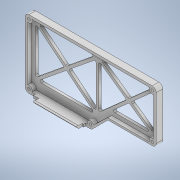
# Autodesk Inventor part: bottom rev3
Saved by Autodesk Inventor 2021 (Build 250183000, 183)
## iProperties
Created: 2024-09-17
Part Number: bottom rev3
Material: Generic
Document SubType Name: Modeling
Designer: Toby
Density: 1 g/cm^3
Appearance: Default
Author: Toby
Autodesk Inventor part; units mm, degrees
ref_plane "YZ Plane" through (0, 0, 0) normal (1, 0, 0) x (0, 1, 0)
ref_plane "XZ Plane" through (0, 0, 0) normal (0, 1, 0) x (-1, 0, 0)
ref_plane "XY Plane" through (0, 0, 0) normal (0, 0, 1) x (1, 0, 0)
sketch "Sketch1" plane through (0, 0, 0) normal (0, 0, 1) x (1, 0, 0)
  line L0 (-50, 26) -> (50, 26)
  line L1 (50, 26) -> (50, -26)
  line L2 (50, -26) -> (-50, -26)
  line L3 (-50, -26) -> (-50, 26)
  point P0 (0, 0)
  dimension "d0" = 52
  dimension "d1" = 100
  dimension "d2" = 26
  dimension "d3" = 50
  constraints: 8 end point, 2 parallel, 1 horizontal, 1 perpendicular
  measures "d0" distance of L2.end L0.start
  measures "d1" distance of L0.start L0.end
  measures "d2" distance from line of point (0, 0) L0
  measures "d3" distance from line of point (0, 0) L3
extrude "Extrusion1" add sketch "Sketch1" along normal blind 2
sketch "Sketch2" plane through (0, 0, 2) normal (0, 0, 1) x (1, 0, 0)
  line L0 (-50, 26) -> (-50, -26) projected
  line L1 (-50, -26) -> (50, -26) projected
  circle A0 centre (-47, 23) radius 1
  circle A1 centre (-47, 23) radius 2.5
  circle A2 centre (-47, -23) radius 1
  circle A3 centre (-47, -23) radius 2.5
  circle A4 centre (0, -23) radius 1
  circle A5 centre (0, -23) radius 2.5
  circle A6 centre (47, 23) radius 1
  circle A7 centre (47, 23) radius 2.5
  circle A8 centre (47, -11) radius 1
  circle A9 centre (47, -11) radius 2.5
  point P0 (0, 0)
  dimension "d6" = 3
  dimension "d7" = 3
  dimension "d8" = 50
  dimension "d9" = 3
  dimension "d10" = 97
  dimension "d11" = 15
  dimension "d12" = 3
  dimension "d13" = 49
  dimension "d14" = 97
  dimension "d15" = 49
  dimension "d16" = 2
  dimension "d17" = 5
  dimension "d18" = 2
  dimension "d19" = 5
  dimension "d20" = 2
  dimension "d21" = 5
  dimension "d22" = 2
  dimension "d23" = 5
  dimension "d24" = 2
  dimension "d25" = 5
  constraints: 10 centre point, 10 coincident
  measures "d6" distance from line of L0 point (-47, -23)
  measures "d7" distance from line of L1 point (-47, -23)
  measures "d8" distance from line of L0 point (0, -23)
  measures "d9" distance from line of L1 point (0, -23)
  measures "d10" distance from line of L0 point (47, -11)
  measures "d11" distance from line of L1 point (47, -11)
  measures "d12" distance from line of L0 point (-47, 23)
  measures "d13" distance from line of L1 point (-47, 23)
  measures "d14" distance from line of L0 point (47, 23)
  measures "d15" distance from line of L1 point (47, 23)
  measures "d16" diameter of A0
  measures "d17" diameter of A1
  measures "d18" diameter of A2
  measures "d19" diameter of A3
  measures "d20" diameter of A4
  measures "d21" diameter of A5
  measures "d22" diameter of A6
  measures "d23" diameter of A7
  measures "d24" diameter of A8
  measures "d25" diameter of A9
extrude "Extrusion2" add sketch "Sketch2" along normal blind 3
sketch "Sketch3" plane through (0, 0, 0) normal (0, 0, -1) x (-1, 0, 0)
  circle A0 centre (-47, 23) radius 1 projected
  circle A1 centre (47, 23) radius 1 projected
  circle A2 centre (47, -23) radius 1 projected
  circle A3 centre (0, -23) radius 1 projected
  circle A4 centre (-47, -11) radius 1 projected
  point P0 (0, 0)
  constraints: 5 coincident
hole "Hole1" at (47, 23, 0) at (-47, 23, 0) at (-47, -23, 0) at (0, -23, 0) at (47, -11, 0) direction (0, 0, 1) diameter 2 depth 10 tip angle 118 countersink diameter 5 countersink angle 90
sketch "Sketch4" plane through (0, 0, 2) normal (0, 0, 1) x (1, 0, 0)
  line L0 (50, -26) -> (50, 26) projected
  line L1 (50, -26) -> (13.1, -26)
  line L2 (13.1, -26) -> (13.1, -13.5)
  line L3 (13.1, -13.5) -> (50, -13.5)
  line L4 (50, -13.5) -> (50, -26)
  line L5 (-50, 26) -> (-50, -26) projected
  point P0 (0, 0)
  dimension "d35" = 12.5
  dimension "d36" = 63.1
  constraints: 8 end point, 2 parallel, 1 horizontal, 1 perpendicular
  measures "d35" distance between parallel lines of L1 L3
  measures "d36" distance between parallel lines of L5 L2
extrude "Extrusion3" cut sketch "Sketch4" against normal blind 3
sketch "Sketch5" plane through (0, 0, 2) normal (0, 0, 1) x (1, 0, 0)
  line L0 (-50, -26) -> (13.1, -26) projected
  line L1 (-50, 26) -> (-50, -26) projected
  line L2 (13.1, -13.5) -> (0.673, -26)
  line L3 (0.673, -26) -> (13.1, -26)
  line L4 (13.1, -26) -> (13.1, -13.5) projected
  line L5 (13.1, -13.5) -> (13.1, -26)
  point P0 (0, 0)
  dimension "d39" = 50.673
  constraints: 6 end point, 1 horizontal, 1 point on line, 1 vertical
  measures "d39" distance from line of L1 L2.end
extrude "Extrusion4" cut sketch "Sketch5" against normal blind 3
sketch "Sketch6" plane through (0, 0, 2) normal (0, 0, 1) x (1, 0, 0)
  line L0 (-50, 26) -> (-50, -26) projected
  line L1 (-50, -26) -> (0.673, -26) projected
  line L2 (-50, 26) -> (-48, 26)
  line L3 (-48, 26) -> (-48, -26)
  line L4 (-48, -26) -> (-50, -26)
  line L5 (-50, -26) -> (-50, 26)
  line L6 (50, -13.5) -> (50, 26) projected
  line L7 (-48, 26) -> (50, 26)
  line L8 (50, 26) -> (50, 24)
  line L9 (50, 24) -> (-48, 24)
  line L10 (-48, 24) -> (-48, 26)
  circle A0 centre (47, -11) radius 2.5 projected
  line L11 (50, 24) -> (48, 24)
  line L12 (48, 24) -> (48, -13.2913)
  line L13 (48, -13.2913) -> (50, -13.2913)
  line L14 (50, -13.2913) -> (50, 24)
  circle A1 centre (0, -23) radius 1 projected
  line L15 (-48, -26) -> (0, -26)
  line L16 (0, -26) -> (0, -24)
  line L17 (0, -24) -> (-48, -24)
  line L18 (-48, -24) -> (-48, -26)
  line L19 (50, -13.5) -> (47, -13.5) projected
  line L20 (50, -13.2913) -> (48, -13.2913)
  line L21 (48, -13.2913) -> (48, -13.5)
  line L22 (48, -13.5) -> (50, -13.5)
  line L23 (50, -13.5) -> (50, -13.2913)
  line L24 (0.673, -26) -> (13.1, -13.5) projected
  line L25 (13.1, -13.5) -> (50, -13.5)
  line L26 (50, -13.5) -> (50, -12)
  line L27 (50, -12) -> (13.1, -12)
  line L28 (13.1, -12) -> (13.1, -13.5)
  line L29 (0, -26) -> (0.673, -26)
  line L30 (0.673, -26) -> (13.1, -13.5)
  line L31 (13.1, -12) -> (13.1, -13.5)
  line L32 (13.1, -12) -> (0.6867, -23.7269)
  line L33 (0.6867, -23.7269) -> (0.6867, -24)
  line L34 (0.6867, -24) -> (0, -24)
  point P0 (0, 0)
  point P1 (44.7087, -12)
  point P2 (-48, 24)
  point P3 (48, -8.7087)
  dimension "d42" = 2
  dimension "d43" = 2
  dimension "d44" = 2
  dimension "d45" = 1.5
  constraints: 60 end point, 13 parallel, 8 perpendicular, 6 horizontal, 6 point on line, 3 point on circle, 2 tangent, 1 collinear
  measures "d42" distance of L3.end L4.end
  measures "d43" distance of L7.end L8.end
  measures "d44" distance of L13.end L12.end
  measures "d45" distance of L26.end L25.end
extrude "Extrusion5" add sketch "Sketch6" along normal blind 3 contours L2 L3 L1 L0 | L7 L6 L9 L3 | L3 L17 L16 L1 | L16 L34 L33 L32 L28 L24 L1 | L9 L6 L27 A0 L12 | L6 L13 A0 L27 | L28 L27 A0 L25 | L6 L19 L21 L13 | A0 L21 L19
fillet "Fillet1" radius 3 4 edges at (50, 26, 2.5) (50, -13.5, 2.5) (-50, -26, 2.5) (-50, 26, 2.5)
sketch "Sketch7" plane through (0, 0, 5) normal (0, 0, 1) x (1, 0, 0)
  line L0 (-47, -26) -> (0.673, -26) projected
  line L1 (-42.4, -26) -> (-3.6, -26)
  line L2 (-3.6, -26) -> (-3.6, -19.3)
  line L3 (-3.6, -19.3) -> (-42.4, -19.3)
  line L4 (-42.4, -19.3) -> (-42.4, -26)
  line L5 (-50, 23) -> (-50, -23) projected
  point P0 (0, 0)
  dimension "d49" = 7.6
  dimension "d50" = 46.4
  dimension "d51" = 6.7
  constraints: 8 end point, 2 parallel, 1 horizontal, 1 perpendicular, 1 point on line
  measures "d49" distance between parallel lines of L5 L4
  measures "d50" distance between parallel lines of L5 L2
  measures "d51" distance between parallel lines of L0 L3
extrude "Extrusion6" cut sketch "Sketch7" against normal blind 3
sketch "Sketch8" plane through (0, 0, 2) normal (0, 0, 1) x (1, 0, 0)
  line L0 (-47, -26) -> (-42.4, -26) projected
  line L1 (-42.4, -26) -> (-37.4, -26)
  line L2 (-37.4, -26) -> (-37.4, -24)
  line L3 (-37.4, -24) -> (-42.4, -24)
  line L4 (-42.4, -24) -> (-42.4, -26)
  point P0 (0, 0)
  dimension "d54" = 5
  dimension "d55" = 2
  constraints: 8 end point, 2 parallel, 1 horizontal, 1 perpendicular
  measures "d54" distance of L2.end L3.end
  measures "d55" distance between parallel lines of L1 L3
extrude "Extrusion7" add sketch "Sketch8" along normal blind 12
sketch "Sketch9" plane through (0, 0, 2) normal (0, 0, 1) x (1, 0, 0)
  line L0 (-39.4, -21.4) -> (-28.4, -21.4)
  line L1 (-28.4, -21.4) -> (-28.4, -22.6)
  line L2 (-28.4, -22.6) -> (-39.4, -22.6)
  line L3 (-39.4, -22.6) -> (-39.4, -21.4)
  line L4 (-37.4, -24) -> (-42.4, -24) projected
  line L5 (-42.4, -24) -> (-42.4, -26) projected
  line L6 (-15.6, -21.4) -> (-3.6, -21.4)
  line L7 (-3.6, -21.4) -> (-3.6, -22.6)
  line L8 (-3.6, -22.6) -> (-15.6, -22.6)
  line L9 (-15.6, -22.6) -> (-15.6, -21.4)
  line L10 (-3.6, -24) -> (-3.6, -26) projected
  line L11 (-2.2913, -24) -> (-3.6, -24) projected
  point P0 (0, 0)
  dimension "d58" = 1.4
  dimension "d59" = 1.2
  dimension "d60" = 3
  dimension "d61" = 14
  dimension "d62" = 1.2
  dimension "d63" = 1.4
  dimension "d64" = 12
  constraints: 16 end point, 4 parallel, 2 horizontal, 2 perpendicular, 1 collinear
  measures "d58" distance between parallel lines of L4 L2
  measures "d59" distance between parallel lines of L2 L0
  measures "d60" distance between parallel lines of L5 L3
  measures "d61" distance between parallel lines of L5 L1
  measures "d62" distance between parallel lines of L8 L6
  measures "d63" distance between parallel lines of L11 L8
  measures "d64" distance of L6.start L6.end
extrude "Extrusion8" add sketch "Sketch9" along normal blind 3
chamfer "Chamfer1" distance 1 angle 45 2 edges at (-33.9, -21.4, 2) (-9.6, -21.4, 2)
sketch "Sketch10" plane through (0, 0, 2) normal (0, 0, 1) x (1, 0, 0)
  line L0 (-3.6, -22.6) -> (-3.6, -21.4) projected
  line L1 (-3.6, -24) -> (-2.2913, -24) projected
  line L2 (-3.6, -21.4) -> (-2.4, -21.4)
  line L3 (-2.4, -21.4) -> (-2.4, -24)
  line L4 (-2.4, -24) -> (-3.6, -24)
  line L5 (-3.6, -24) -> (-3.6, -21.4)
  line L6 (-2.4, -24) -> (-2.1404, -24)
  line L7 (-2.1404, -24) -> (-2.1404, -23.6677)
  line L8 (-2.1404, -23.6677) -> (-2.4, -23.6677)
  line L9 (-2.4, -23.6677) -> (-2.4, -24)
  point P0 (0, 0)
  dimension "d70" = 1.2
  constraints: 16 end point, 4 parallel, 2 horizontal, 2 perpendicular, 1 point on line
  measures "d70" distance of L3.end L4.end
extrude "Extrusion9" add sketch "Sketch10" along normal blind 3
fillet "Fillet2" radius 1 1 edges at (-2.4, -21.4, 3.5)
sketch "Sketch12" plane through (0.673, -26, 0) normal (0, -1, 0) x (1, 0, 0)
  line L0 (-43.073, 5) -> (-43.073, 14) projected
  line L1 (-43.073, 14) -> (-38.073, 14)
  line L2 (-38.073, 14) -> (-38.073, 5)
  line L3 (-38.073, 5) -> (-43.073, 5)
  line L4 (-43.073, 5) -> (-43.073, 14)
  line L5 (-38.073, 2) -> (-38.073, 14) projected
  line L6 (-40.073, 5) -> (-29.073, 5) projected
  point P0 (-0.673, 0)
  constraints: 8 end point, 2 collinear, 2 parallel, 1 horizontal, 1 perpendicular
extrude "Extrusion11" cut sketch "Sketch12" against normal blind 3
sketch "Sketch13" plane through (0, 0, 2) normal (0, 0, 1) x (1, 0, 0)
  line L0 (-45, 21) -> (45, 21)
  line L1 (45, 21) -> (45, -9)
  line L2 (45, -9) -> (-45, -9)
  line L3 (-45, -9) -> (-45, 21)
  line L4 (-45, -9) -> (2, -9)
  line L5 (2, -9) -> (2, -17.4)
  line L6 (2, -17.4) -> (-45, -17.4)
  line L7 (-45, -17.4) -> (-45, -9)
  line L8 (-44.7087, 24) -> (44.7087, 24) projected
  line L9 (-48, -20.7087) -> (-48, 20.7087) projected
  line L10 (48, 20.7087) -> (48, -8.7087) projected
  line L11 (44.7087, 24) -> (-44.7087, 24) projected
  line L12 (48, -8.7087) -> (48, 20.7087) projected
  line L13 (44, 24) -> (48, 24)
  line L14 (48, 24) -> (48, 20)
  line L15 (48, 20) -> (44, 20)
  line L16 (44, 20) -> (44, 24)
  circle A0 centre (47, 23) radius 1 projected
  line L17 (44.7087, -12) -> (13.1, -12) projected
  line L18 (-28.4, -20.4) -> (-39.4, -20.4) projected
  line L19 (50, -10.5) -> (50, 23) projected
  point P0 (0, 0)
  point P1 (48, 24)
  point P2 (45, 20)
  point P3 (44, 21)
  dimension "d79" = 3
  dimension "d80" = 3
  dimension "d81" = 3
  dimension "d82" = 3
  dimension "d83" = 3
  dimension "d84" = 3
  dimension "d85" = 3
  dimension "d86" = 48
  constraints: 24 end point, 6 parallel, 3 horizontal, 3 perpendicular, 2 point on line
  measures "d79" distance between parallel lines of L0 L8
  measures "d80" distance between parallel lines of L9 L3
  measures "d81" distance between parallel lines of L10 L1
  measures "d82" distance from line of A0.centre L16
  measures "d83" distance from line of L15 A0.centre
  measures "d84" distance between parallel lines of L17 L2
  measures "d85" distance between parallel lines of L18 L6
  measures "d86" distance between parallel lines of L19 L5
extrude "Extrusion12" cut sketch "Sketch13" against normal blind 2 contours L0 L16 L15 L1 L2 L3 | L2 L5 L6 L7
chamfer "Chamfer2" distance 8.4 angle 45 1 edges at (2, -9, 1)
sketch "Sketch14" plane through (0, 0, 5) normal (0, 0, 1) x (1, 0, 0)
  line L0 (-28.4, -20.4) -> (-39.4, -20.4) projected
  line L1 (-39.4, -20.4) -> (-2.4, -20.4)
  line L2 (-2.4, -20.4) -> (-2.4, -24)
  line L3 (-2.4, -24) -> (-39.4, -24)
  line L4 (-39.4, -24) -> (-39.4, -20.4)
  line L5 (-37.4, -24) -> (-44.7087, -24) projected
  line L6 (-3.6, -22.6) -> (-3.6, -26) projected
  point P0 (0, 0)
  dimension "d92" = 1.2
  constraints: 8 end point, 2 parallel, 1 collinear, 1 horizontal, 1 perpendicular
  measures "d92" distance between parallel lines of L6 L2
extrude "Extrusion13" cut sketch "Sketch14" against normal blind 3
sketch "Sketch15" plane through (0, 0, 5) normal (0, 0, 1) x (1, 0, 0)
  line L0 (-44.7087, -24) -> (-37.4, -24) projected
  line L1 (-42.4, -24) -> (-3.6, -24)
  line L2 (-3.6, -24) -> (-3.6, -26)
  line L3 (-3.6, -26) -> (-42.4, -26)
  line L4 (-42.4, -26) -> (-42.4, -24)
  line L5 (-3.6, -26) -> (-37.4, -26) projected
  line L6 (-50, 23) -> (-50, -23) projected
  line L7 (-3.6, -24) -> (-3.6, -26) projected
  point P0 (0, 0)
  dimension "d95" = 7.6
  constraints: 8 end point, 2 collinear, 2 parallel, 1 horizontal, 1 perpendicular, 1 point on line
  measures "d95" distance between parallel lines of L6 L4
extrude "Extrusion14" cut sketch "Sketch15" against normal blind 5
sketch "Sketch16" plane through (0, 0, 2) normal (0, 0, 1) x (1, 0, 0)
  line L0 (-45, -17.4) -> (-45, 21) projected
  line L1 (-45, 21) -> (2.1434, -17.4) construction
  line L2 (-45.6315, 20.2247) -> (1.5119, -18.1753)
  line L3 (2.775, -16.6247) -> (-44.3685, 21.7753)
  arc A0 (-44.3685, 21.7753) -> (-45.6315, 20.2247) centre (-45, 21) ccw
  arc A1 (1.5119, -18.1753) -> (2.775, -16.6247) centre (2.1434, -17.4) ccw
  line L4 (2, -17.4) -> (-45, -17.4) projected
  line L5 (-45, -17.4) -> (2.1434, 21) construction
  line L6 (44, 21) -> (-45, 21) projected
  line L7 (-44.3685, -18.1753) -> (2.775, 20.2247)
  line L8 (1.5119, 21.7753) -> (-45.6315, -16.6247)
  arc A2 (-45.6315, -16.6247) -> (-44.3685, -18.1753) centre (-45, -17.4) ccw
  arc A3 (2.775, 20.2247) -> (1.5119, 21.7753) centre (2.1434, 21) ccw
  line L9 (2.1434, 21) -> (2.1434, -17.4) construction
  line L10 (1.1434, 21) -> (1.1434, -17.4)
  line L11 (3.1434, -17.4) -> (3.1434, 21)
  arc A4 (3.1434, 21) -> (1.1434, 21) centre (2.1434, 21) ccw
  arc A5 (1.1434, -17.4) -> (3.1434, -17.4) centre (2.1434, -17.4) ccw
  line L12 (45, -9) -> (10.4, -9) projected
  line L13 (2.1434, 21) -> (45, -9) construction
  line L14 (1.57, 20.1808) -> (44.4265, -9.8192)
  line L15 (45.5735, -8.1808) -> (2.7169, 21.8192)
  arc A6 (2.7169, 21.8192) -> (1.57, 20.1808) centre (2.1434, 21) ccw
  arc A7 (44.4265, -9.8192) -> (45.5735, -8.1808) centre (45, -9) ccw
  line L16 (44, 20) -> (2.1434, -17.2566) construction
  line L17 (10.4, -9) -> (2, -17.4) projected
  line L18 (43.3351, 20.747) -> (1.4786, -16.5096)
  line L19 (2.8083, -18.0035) -> (44.6649, 19.253)
  arc A8 (44.6649, 19.253) -> (43.3351, 20.747) centre (44, 20) ccw
  arc A9 (1.4786, -16.5096) -> (2.8083, -18.0035) centre (2.1434, -17.2566) ccw
  point P0 (0, 0)
  point P1 (-21.4283, 1.8)
  point P2 (-21.4283, 1.8)
  point P3 (2.1434, 1.8)
  point P4 (23.5717, 6)
  point P5 (23.0717, 1.3717)
  point P6 (-19.8449, 1.8)
  point P7 (1.1434, 18.8957)
  point P8 (1.1434, -15.2957)
  point P9 (24.5929, 4.0645)
  point P10 (3.1434, -15.0277)
  point P11 (3.1434, 19.0793)
  point P12 (-21.4283, 3.0898)
  point P13 (-23.0117, 1.8)
  point P14 (-21.4283, 0.5102)
  point P15 (3.0734, -17.7675)
  point P16 (26.2768, 2.8858)
  point P17 (27.8121, 4.2524)
  point P18 (26.1282, 5.4311)
  dimension "d98" = 2
  dimension "d99" = 2
  dimension "d100" = 2
  dimension "d101" = 2
  dimension "d102" = 2
  constraints: 40 end point, 20 point on circle, 20 tangent, 10 centre point, 5 midpoint, 5 parallel, 5 point on line, 1 concentric, 1 perpendicular
  measures "d98" diameter of A1
  measures "d99" diameter of A3
  measures "d100" diameter of A5
  measures "d101" diameter of A7
  measures "d102" diameter of A9
extrude "Extrusion15" add sketch "Sketch16" against normal blind 2 contours L4 L7 A2 L8 L0 | L0 L8 L2 L7 L4 | L2 A0 L3 L6 L0 | L0 L6 L3 L8 L2 | L8 L3 L7 L2 | L4 A5 L2 | L2 L7 L3 L10 L4 | L8 L6 L10 L7 L3 | A5 L4 A9 L19 A1 | L10 A9 L4 | L8 A4 L6 | L19 A9 L4 L17 A1 | A1 L11 L17 L12 L19 | A9 L18 L3 L17 L4 | L10 L3 L18 A9 | L10 L7 L14 L11 L18 L3 | L10 A6 L14 L7 | A4 A3 L6 | L6 A3 L7 L14 A6 | A1 L17 L11 | L12 L17 L11 L18 L14 L19 | L18 L11 L17 L3 | L7 A3 L11 L14 | A3 L15 L6 | L6 L15 L18 L14 L11 | L14 L19 L15 A7 | L14 L18 L15 L19 | L15 L18 A8 L19
fillet "Fillet3" radius 1 12 edges at (-45, -16.1102, 1) (-43.4166, -17.4, 1) (0.56, -17.4, 1) (-21.4283, 0.5102, 1) (-21.4283, 3.0898, 1) (-23.0117, 1.8, 1) (-19.8449, 1.8, 1) (-45, 19.7102, 1) (-43.4166, 21, 1) (0.56, 21, 1) (1.1434, 18.8957, 1) (1.1434, -15.2957, 1)
fillet "Fillet4" radius 1 11 edges at (43.2562, -9, 1) (45, -7.7793, 1) (27.8121, 4.2524, 1) (26.2768, 2.8858, 1) (24.5929, 4.0645, 1) (26.1282, 5.4311, 1) (12.9235, -9, 1) (3.1434, -15.0277, 1) (3.1434, 19.0793, 1) (44, 21, 1) (3.8872, 21, 1)
sketch "Sketch17" plane through (0, 0, 0) normal (0, 0, -1) x (-1, 0, 0)
  arc A0 (-47, -13.5) -> (-44.7258, -9.9617) centre (-47, -11) ccw projected
  circle A1 centre (47, 23) radius 1 projected
  point P0 (0, 0)
  constraints: 2 coincident
hole "Hole2" at (47, -11, 0) at (-47, 23, 0) direction (0, 0, 1) diameter 2 depth 4 tip angle 118 countersink diameter 5 countersink angle 90
sketch "Sketch23" plane through (-47, -26, 0) normal (0, -1, 0) x (1, 0, 0)
  line L0 (4.6, 0) -> (43.4, 0)
  line L1 (43.4, 0) -> (43.4, 6.5)
  line L2 (43.4, 6.5) -> (4.6, 6.5)
  line L3 (4.6, 6.5) -> (4.6, 0)
  line L4 (4.6, 0) -> (4.6, 5) projected
  line L5 (43.4, 5) -> (43.4, 0) projected
  line L6 (43.4, 0) -> (4.6, 0) projected
  line L7 (0, 0) -> (4.6, 0) projected
  line L8 (0, 5) -> (4.6, 5) projected
  point P0 (47, 0)
  dimension "d146" = 6.5
  dimension "d147" = 5
  constraints: 8 end point, 3 collinear, 2 parallel, 1 horizontal, 1 perpendicular
  measures "d146" distance between parallel lines of L0 L2
  measures "d147" distance between parallel lines of L7 L8
extrude "Extrusion20" add sketch "Sketch23" against normal blind 2
sketch "Sketch24" plane through (0.673, -26, 0) normal (0, -1, 0) x (1, 0, 0)
  line L0 (-43.073, 5) -> (-43.073, 6.5) projected
  line L1 (-43.073, 6.5) -> (-4.273, 6.5) projected
  line L2 (-43.073, 5) -> (-42.773, 5)
  line L3 (-42.773, 5) -> (-42.773, 6.5)
  line L4 (-42.773, 6.5) -> (-43.073, 6.5)
  line L5 (-43.073, 6.5) -> (-43.073, 5)
  line L6 (-4.273, 5) -> (-4.273, 6.5) projected
  line L7 (-4.273, 5) -> (-4.573, 5)
  line L8 (-4.573, 5) -> (-4.573, 6.5)
  line L9 (-4.573, 6.5) -> (-4.273, 6.5)
  line L10 (-4.273, 6.5) -> (-4.273, 5)
  point P0 (-0.673, 0)
  dimension "d150" = 0.3
  dimension "d151" = 0.3
  constraints: 16 end point, 4 parallel, 2 horizontal, 2 perpendicular, 2 point on line
  measures "d150" distance between parallel lines of L0 L3
  measures "d151" distance between parallel lines of L6 L8
extrude "Extrusion21" cut sketch "Sketch24" against normal blind 2
fillet "Fillet5" radius 3 1 edges at (0.673, -26, 2.5)
sketch "Sketch25" plane through (0, 0, 2) normal (0, 0, 1) x (1, 0, 0)
  arc A0 (44.6649, 19.253) -> (45, 20) centre (44, 20) ccw projected
  line L0 (44, 20) -> (46, 20)
  line L1 (46, 20) -> (46, 18)
  line L2 (46, 18) -> (44, 18)
  line L3 (44, 18) -> (44, 20)
  circle A1 centre (44, 18) radius 1
  point P0 (0, 0)
  point P1 (44, 19)
  point P2 (45, 18)
  dimension "d155" = 2
  dimension "d156" = 2
  dimension "d157" = 2
  constraints: 8 end point, 2 parallel, 1 centre point, 1 coincident, 1 horizontal, 1 perpendicular
  measures "d155" distance of L1.end L2.end
  measures "d156" distance of L0.end L1.end
  measures "d157" diameter of A1
extrude "Extrusion22" add sketch "Sketch25" against normal blind 2 contours L0 L1 L2 A1 L3
sketch "Sketch26" plane through (-47, -26, 0) normal (0, -1, 0) x (1, 0, 0)
  line L0 (43.1, 6.5) -> (4.9, 6.5) projected
  line L1 (9, 6.5) -> (42.2, 6.5)
  line L2 (42.2, 6.5) -> (42.2, 9.311)
  line L3 (42.2, 9.311) -> (9, 9.311)
  line L4 (9, 9.311) -> (9, 6.5)
  line L5 (4.9, 5) -> (0, 5) projected
  line L6 (-3, 5) -> (-3, 0) projected
  point P0 (47, 0)
  point P1 (42.2, 6.5)
  dimension "d160" = 1.5
  dimension "d161" = 2.811
  dimension "d162" = 12
  dimension "d163" = 33.2
  constraints: 8 end point, 2 parallel, 1 horizontal, 1 perpendicular, 1 point on line
  measures "d160" distance between parallel lines of L5 L0
  measures "d161" distance between parallel lines of L0 L3
  measures "d162" distance between parallel lines of L6 L4
  measures "d163" distance of L2.end L3.end
extrude "Extrusion23" add sketch "Sketch26" against normal blind 2
sketch "Sketch27" plane through (-38, -26, 6.5) normal (-1, 0, 0) x (0, 0, 1)
  line L0 (2.811, 0) -> (2.811, 2) projected
  line L1 (2.811, 0) -> (4.47, 1.9772)
  line L2 (2.811, 0) -> (5.392, 0) construction
  line L3 (4.47, 1.9772) -> (2.9379, 3.2627)
  line L4 (2.9379, 3.2627) -> (1.8784, 2)
  line L5 (0, 2) -> (2.811, 2) projected
  point P0 (-6.5, 26)
  dimension "d166" = 2.581
  dimension "d167" = 50
  dimension "d168" = 2
  constraints: 8 end point, 2 perpendicular, 1 equal length, 1 horizontal, 1 point on line
  measures "d166" distance of L0.start L1.end
  measures "d167" angle of L2 L1
  measures "d168" distance of L1.end L3.end
extrude "Extrusion24" add sketch "Sketch27" against normal blind 33.2
sketch "Sketch28" plane through (-38, -26, 6.5) normal (-1, 0, 0) x (0, 0, 1)
  line L0 (2.9379, 3.2627) -> (4.47, 1.9772) projected
  line L1 (3.5508, 2.7485) -> (2.9227, 2)
  line L2 (1.8784, 2) -> (2.9379, 3.2627) projected
  line L3 (2.9227, 2) -> (1.8784, 2)
  line L4 (1.8784, 2) -> (2.9379, 3.2627)
  line L5 (2.9379, 3.2627) -> (3.5508, 2.7485)
  line L6 (2.811, 0) -> (4.47, 1.9772) projected
  line L7 (0, 2) -> (1.8784, 2) projected
  point P0 (-6.5, 26)
  dimension "d171" = 1.2
  constraints: 8 end point, 2 collinear, 2 perpendicular, 1 horizontal, 1 point on line
  measures "d171" distance between parallel lines of L6 L1
extrude "Extrusion25" cut sketch "Sketch28" against normal blind 33.2
sketch "Sketch29" plane through (-47, -26, 0) normal (0, -1, 0) x (1, 0, 0)
  line L0 (9, 10.97) -> (9, 10.0508) projected
  line L1 (9, 10.97) -> (9.1, 10.97)
  line L2 (9.1, 10.97) -> (9.1, 6.5)
  line L3 (9.1, 6.5) -> (9, 6.5)
  line L4 (9, 6.5) -> (9, 10.97)
  line L5 (42.2, 10.97) -> (42.1, 10.97)
  line L6 (42.1, 10.97) -> (42.1, 6.5)
  line L7 (42.1, 6.5) -> (42.2, 6.5)
  line L8 (42.2, 6.5) -> (42.2, 10.97)
  line L9 (42.2, 6.5) -> (42.2, 9.311) projected
  line L10 (43.1, 6.5) -> (42.2, 6.5) projected
  line L11 (9, 6.5) -> (4.9, 6.5) projected
  point P0 (47, 0)
  point P1 (9, 10.0508)
  dimension "d174" = 0.1
  dimension "d175" = 0.1
  constraints: 16 end point, 4 parallel, 3 collinear, 2 horizontal, 2 perpendicular, 1 point on line
  measures "d174" distance between parallel lines of L4 L2
  measures "d175" distance between parallel lines of L8 L6
extrude "Extrusion26" cut sketch "Sketch29" against normal blind 5
body "Solid1"
